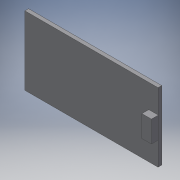
# Autodesk Inventor part: ESP
Saved by Autodesk Inventor 2019 (Build 230136000, 136)
## iProperties
Created: 2021-03-14
Part Number: ESP
Material: Generic
Document SubType Name: Modeling
Designer: Vijay
Density: 1 g/cm^3
Appearance: Default
Author: Vijay
Autodesk Inventor part; units mm, degrees
ref_plane "YZ Plane" through (0, 0, 0) normal (1, 0, 0) x (0, 1, 0)
ref_plane "XZ Plane" through (0, 0, 0) normal (0, 1, 0) x (-1, 0, 0)
ref_plane "XY Plane" through (0, 0, 0) normal (0, 0, 1) x (1, 0, 0)
sketch "Sketch1" plane through (0, 0, 0) normal (0, 0, 1) x (1, 0, 0)
  line L0 (-27.2487, 18.9041) -> (30.7513, 18.9041)
  line L1 (30.7513, 18.9041) -> (30.7513, -11.0959)
  line L2 (30.7513, -11.0959) -> (-27.2487, -11.0959)
  line L3 (-27.2487, -11.0959) -> (-27.2487, 18.9041)
  point P0 (0, 0)
  dimension "d0" = 58
  dimension "d1" = 30
  constraints: 8 end point, 2 parallel, 1 horizontal, 1 perpendicular
  measures "d0" distance of L0.start L0.end
  measures "d1" distance of L2.end L0.start
extrude "Extrusion1" add sketch "Sketch1" along normal blind 1.6
sketch "Sketch2" plane through (0, 0, 1.6) normal (0, 0, 1) x (1, 0, 0)
  line L0 (-27.2487, 18.9041) -> (-27.2487, -11.0959) projected
  line L1 (-33.3397, 3.9041) -> (37.3042, 3.9041)
  line L2 (30.862, 8.6066) -> (26.7324, 8.6066)
  line L3 (26.7324, 8.6066) -> (26.7324, -0.7984)
  line L4 (26.7324, -0.7984) -> (30.862, -0.7984)
  line L5 (30.862, -0.7984) -> (30.862, 8.6066)
  point P0 (0, 0)
  constraints: 10 end point, 2 horizontal, 2 parallel, 1 perpendicular, 1 other
extrude "Extrusion2" add sketch "Sketch2" along normal blind 3
body "Solid1"
